Autodesk Inventor part; units mm, degrees
(part 2 of 2)
sketch "스케치31" plane through (8, 0, 0) normal (1, 0, 0) x (0, 0, -1)
  line L0 (56, 75.2541) -> (56.1, 75.2268) projected
  line L1 (56, 75.2541) -> (56, 75.2541) projected
  line L2 (56.1, 75.2268) -> (56, 75.2541) projected
  line L3 (56.1, 75.2268) -> (56.1, 75.2268) projected
  line L4 (50, 72.5) -> (50, 75.5) projected
  line L5 (56, 65.5) -> (56, 62.5) projected
  line L6 (50, 62.5) -> (50, 65.5) projected
  line L7 (46.8062, 25.5) -> (46.8062, 25.5) projected
  line L8 (46.8062, 25.5) -> (46.8062, 25.5) projected
  line L9 (45.4221, 28.5) -> (45.4221, 28.5) projected
  line L10 (45.4221, 28.5) -> (45.4221, 28.5) projected
  line L11 (41.5966, 28.9171) -> (43.8593, 31.1798) projected
  line L12 (38.9095, 21.9874) -> (36.6468, 19.7247) projected
  line L13 (34.5255, 21.846) -> (36.7882, 24.1087) projected
  line L14 (26.1876, 8.1912) -> (24.0225, 6.9412) projected
  line L15 (21.0225, 12.1374) -> (23.1876, 13.3874) projected
  line L16 (17.5008, 3.0604) -> (17.5008, 3.0604) projected
  line L17 (17.5008, 3.0604) -> (17.5008, 3.0604) projected
  line L18 (15.0184, 3) -> (15.0184, 3) projected
  line L19 (15.0184, 3) -> (15.0184, 3) projected
  line L20 (14.1878, 6.1) -> (14.1878, 6.1) projected
  line L21 (14.5063, 4.9111) -> (14.1878, 6.1) projected
  line L22 (14.5063, 4.9111) -> (14.5063, 4.9111) projected
  line L23 (14.1878, 6.1) -> (14.5063, 4.9111) projected
  line L24 (12.3623, 7.1374) -> (14.5274, 8.3874) projected
  line L25 (15.25, 0) -> (12.75, 0) projected
  line L26 (15.0184, 3) -> (15.0184, 3) projected
  line L27 (15.0184, 3) -> (15.0184, 3) projected
  line L28 (85.75, 3) -> (88.25, 3) projected
  line L29 (88.25, 0) -> (85.75, 0) projected
  line L30 (158.75, 3) -> (161.25, 3) projected
  line L31 (161.25, 0) -> (158.75, 0) projected
  line L32 (231.75, 3) -> (234.25, 3) projected
  line L33 (234.25, 0) -> (231.75, 0) projected
  line L34 (307.25, 0) -> (304.75, 0) projected
  line L35 (304.9816, 3) -> (304.9816, 3) projected
  line L36 (304.9816, 3) -> (304.9816, 3) projected
  line L37 (302.4992, 3.0604) -> (302.4992, 3.0604) projected
  line L38 (302.4992, 3.0604) -> (302.4992, 3.0604) projected
  line L39 (305.4937, 4.9111) -> (305.4937, 4.9111) projected
  line L40 (305.8122, 6.1) -> (305.4937, 4.9111) projected
  line L41 (305.8122, 6.1) -> (305.8122, 6.1) projected
  line L42 (305.4937, 4.9111) -> (305.8122, 6.1) projected
  line L43 (304.9816, 3) -> (304.9816, 3) projected
  line L44 (304.9816, 3) -> (304.9816, 3) projected
  line L45 (305.4726, 8.3874) -> (307.6377, 7.1374) projected
  line L46 (295.9775, 6.9412) -> (293.8124, 8.1912) projected
  line L47 (296.8124, 13.3874) -> (298.9775, 12.1374) projected
  line L48 (283.3389, 19.739) -> (281.0762, 22.0017) projected
  line L49 (283.1975, 24.123) -> (285.4602, 21.8603) projected
  line L50 (273.1938, 25.5) -> (273.1938, 25.5) projected
  line L51 (273.1938, 25.5) -> (273.1938, 25.5) projected
  line L52 (274.5779, 28.5) -> (274.5779, 28.5) projected
  line L53 (274.5779, 28.5) -> (274.5779, 28.5) projected
  line L54 (276.1264, 31.1941) -> (278.3892, 28.9313) projected
  line L55 (264, 62.5) -> (264, 65.5) projected
  line L56 (270, 65.5) -> (270, 62.5) projected
  line L57 (264, 75.2541) -> (263.9, 75.2268) projected
  line L58 (264, 75.2541) -> (264, 75.2541) projected
  line L59 (263.9, 75.2268) -> (264, 75.2541) projected
  line L60 (263.9, 75.2268) -> (263.9, 75.2268) projected
  line L61 (270, 75.5) -> (270, 72.5) projected
  arc A0 (50, 73.3386) -> (50, 74.6614) centre (49.25, 74) ccw
  arc A1 (50, 63.3386) -> (50, 64.6614) centre (49.25, 64) ccw
  arc A2 (42.2602, 29.5807) -> (43.1956, 30.5161) centre (42.1976, 30.5788) ccw
  arc A3 (35.1891, 22.5097) -> (36.1246, 23.4451) centre (35.1265, 23.5077) ccw
  arc A4 (21.5323, 12.4317) -> (22.6779, 13.0931) centre (21.7301, 13.4119) ccw
  arc A5 (12.872, 7.4317) -> (14.0176, 8.0931) centre (13.0698, 8.4119) ccw
  arc A6 (14.6614, 0) -> (13.3386, 0) centre (14, -0.75) ccw
  arc A7 (87.6614, 0) -> (86.3386, 0) centre (87, -0.75) ccw
  arc A8 (160.6614, 0) -> (159.3386, 0) centre (160, -0.75) ccw
  arc A9 (233.6614, 0) -> (232.3386, 0) centre (233, -0.75) ccw
  arc A10 (306.6614, 0) -> (305.3386, 0) centre (306, -0.75) ccw
  arc A11 (305.9824, 8.0931) -> (307.128, 7.4317) centre (306.9302, 8.4119) ccw
  arc A12 (297.3221, 13.0931) -> (298.4677, 12.4317) centre (298.2699, 13.4119) ccw
  arc A13 (283.8612, 23.4594) -> (284.7966, 22.5239) centre (284.8592, 23.522) ccw
  arc A14 (276.7901, 30.5304) -> (277.7255, 29.595) centre (277.7881, 30.593) ccw
  arc A15 (270, 64.6614) -> (270, 63.3386) centre (270.75, 64) ccw
  arc A16 (270, 74.6614) -> (270, 73.3386) centre (270.75, 74) ccw
  point P0 (0, 0)
  dimension "d326" = 2
  dimension "d327" = 2
  dimension "d328" = 2
  dimension "d329" = 2
  dimension "d330" = 2
  dimension "d331" = 2
  dimension "d332" = 2
  dimension "d333" = 2
  dimension "d334" = 2
  dimension "d335" = 2
  dimension "d336" = 2
  dimension "d337" = 2
  dimension "d338" = 2
  dimension "d339" = 2
  dimension "d340" = 2
  dimension "d341" = 2
  dimension "d342" = 2
  dimension "d343" = 0.75
  dimension "d344" = 0.75
  dimension "d345" = 0.75
  dimension "d346" = 0.75
  dimension "d347" = 0.75
  dimension "d348" = 0.75
  dimension "d349" = 0.75
  dimension "d350" = 0.75
  dimension "d351" = 0.75
  dimension "d352" = 0.75
  dimension "d353" = 0.75
  dimension "d354" = 0.75
  dimension "d355" = 0.75
  dimension "d356" = 0.75
  dimension "d357" = 0.75
  dimension "d358" = 0.75
  dimension "d359" = 0.75
  constraints: 34 point on circle, 34 point on line, 17 centre point
  measures "d326" diameter of A0
  measures "d327" diameter of A1
  measures "d328" diameter of A2
  measures "d329" diameter of A3
  measures "d330" diameter of A4
  measures "d331" diameter of A5
  measures "d332" diameter of A6
  measures "d333" diameter of A7
  measures "d334" diameter of A8
  measures "d335" diameter of A9
  measures "d336" diameter of A10
  measures "d337" diameter of A11
  measures "d338" diameter of A12
  measures "d339" diameter of A13
  measures "d340" diameter of A14
  measures "d341" diameter of A15
  measures "d342" diameter of A16
  measures "d343" distance from line of L4 A0.centre
  measures "d344" distance from line of L6 A1.centre
  measures "d345" distance from line of L11 A2.centre
  measures "d346" distance from line of L13 A3.centre
  measures "d347" distance from line of L15 A4.centre
  measures "d348" distance from line of L24 A5.centre
  measures "d349" distance from line of L25 A6.centre
  measures "d350" distance from line of L29 A7.centre
  measures "d351" distance from line of A8.centre L31
  measures "d352" distance from line of A9.centre L33
  measures "d353" distance from line of A10.centre L34
  measures "d354" distance from line of L45 A11.centre
  measures "d355" distance from line of L47 A12.centre
  measures "d356" distance from line of L49 A13.centre
  measures "d357" distance from line of L54 A14.centre
  measures "d358" distance from line of L56 A15.centre
  measures "d359" distance from line of L61 A16.centre
extrude "돌출40" cut sketch "스케치31" against normal blind 8
